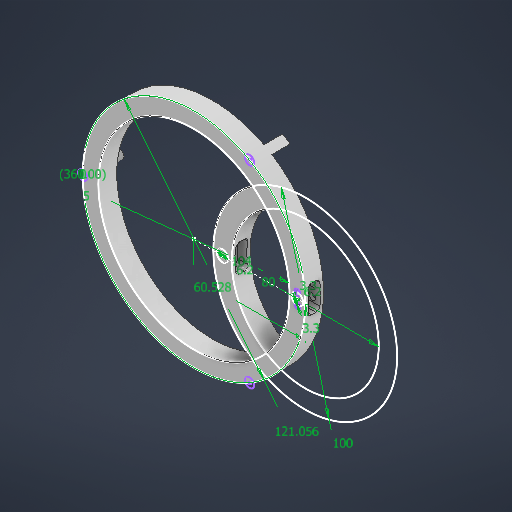
# Autodesk Inventor part: Part4
Saved by Autodesk Inventor 2026.2 (Build 302298000, 298)
## iProperties
Created: 2026-01-26
Part Number: Part4
Material: Generic
Document SubType Name: Modeling
Designer: Cobble
Density: 1 g/cm^3
Appearance: Default
Author: Cobble
Autodesk Inventor part; units mm, degrees
ref_plane "YZ Plane" through (0, 0, 0) normal (1, 0, 0) x (0, 1, 0)
ref_plane "XZ Plane" through (0, 0, 0) normal (0, 1, 0) x (-1, 0, 0)
sketch "Sketch4" plane through (0, 0, 0) normal (0, 1, 0) x (-1, 0, 0)
  circle A0 centre (0, 0) radius 60.528
  line L0 (-60.528, 0) -> (0, 0) construction
  circle A1 centre (0, 0) radius 52
  circle A2 centre (-60.528, 0) radius 50
  circle A3 centre (-60.528, 0) radius 40
  line L1 (-10.528, 0) -> (-20.528, 0) construction
  line L2 (-52, 0) -> (-60.528, 0) construction
  circle A4 centre (-15.528, 0) radius 3.1
  circle A5 centre (-56.264, 0) radius 3.1
  circle A6 centre (-56.264, -3.1) radius 1.65
  circle A7 centre (-56.264, 3.1) radius 1.65
  circle A8 centre (60.528, 0) radius 2.5
  circle A9 centre (-30.264, 52.4188) radius 2.5
  circle A10 centre (-30.264, -52.4188) radius 2.5
  line L3 (60.528, 0) -> (60.528, 0)
  point P0 (-39.3837, 33.9547)
  point P1 (-39.3837, -33.9547)
  point P2 (-31.9492, 41.0274)
  point P3 (-31.9492, -41.0274)
  point P4 (-28.0736, 53.6238)
  point P5 (-32.4028, 51.1243)
  point P6 (60.4764, 2.4995)
  point P7 (60.4764, -2.4995)
  point P8 (-32.4028, -51.1243)
  point P9 (-28.0736, -53.6238)
  dimension "d18" = 104
  dimension "d19" = 80
  dimension "d20" = 121.056
  dimension "d21" = 100
  dimension "d17" = 60.528
  dimension "d29" = 6.2
  dimension "d30" = 6.2
  dimension "d36" = 3.3
  dimension "d37" = 3.3
  dimension "d38" = 5
  dimension "d42" = 360
  dimension "d46" = 0
  constraints: 8 end point, 7 centre point, 4 coincident, 3 point on line, 2 horizontal, 2 midpoint, 2 point on circle, 1 collinear, 19 other
  measures "d17" distance of L0.start L0.end
  measures "d29" diameter of A4
  measures "d30" diameter of A5
  measures "d36" diameter of A6
  measures "d37" diameter of A7
  measures "d38" diameter of A8
  measures "d46" distance of L3.start L3.end
extrude "Extrusion3" add sketch "Sketch4" along normal blind 10 contours A0 A8 | A8 A0 A10 A2 A1 A9 | A9 A0 | A0 A10 | A2 A1 A3 A0 | A0 A3 A1 A2 | A3 A1 A0 | A2 A1 A3 | A4 | A5 A6 A7 picked at (59.7455, 0.5696) picked at (-29.7736, 51.7403) picked at (-29.7736, -51.7403)
ref_plane "Work Plane5" through (60.528, 0, 0) normal (1, 0, 0) x (0, 1, 0)
sketch "Sketch6" plane through (60.528, 0, 0) normal (1, 0, 0) x (0, 1, 0)
  line L0 (10, -60.528) -> (10, 60.528) projected
  line L1 (0, -60.528) -> (0, 60.528) projected
  line L2 (10, -60.528) -> (10, 60.528) projected
  line L3 (10, 0) -> (0, 0)
  line L4 (1.75, 5.5) -> (1.75, -5.5)
  line L5 (3.75, -7.5) -> (6.25, -7.5)
  line L6 (8.25, -5.5) -> (8.25, 5.5)
  line L7 (6.25, 7.5) -> (3.75, 7.5)
  line L8 (1.75, 7.5) -> (8.25, -7.5) construction
  line L9 (1.75, -7.5) -> (8.25, 7.5) construction
  arc A0 (6.25, -7.5) -> (8.25, -5.5) centre (6.25, -5.5) ccw
  arc A1 (1.75, -5.5) -> (3.75, -7.5) centre (3.75, -5.5) ccw
  arc A2 (8.25, 5.5) -> (6.25, 7.5) centre (6.25, 5.5) ccw
  arc A3 (3.75, 7.5) -> (1.75, 5.5) centre (3.75, 5.5) ccw
  point P0 (5, 0)
  dimension "d31" = 15
  dimension "d32" = 6.5
  dimension "d33" = 2
  constraints: 14 end point, 8 point on circle, 8 point on line, 8 tangent, 4 centre point, 4 midpoint, 3 equal radius, 3 perpendicular, 2 parallel
  measures "d31" distance of L8.start L9.start
  measures "d32" distance of L8.end L9.start
  measures "d33" radius of A0
extrude "Extrusion4" cut sketch "Sketch6" against normal blind 45
extrude "Extrusion5" add sketch "Sketch4" along normal blind 20 contours A0 A8 | A9 A0 | A0 A10 picked at (59.7455, 0.5696) picked at (-29.7736, 51.7403) picked at (-29.7736, -51.7403)
body "Solid2"
